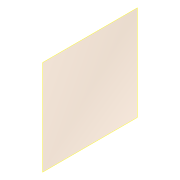
# Autodesk Inventor part: maskBodySolid
Saved by Autodesk Inventor 2018 (Build 220112000, 112)
## iProperties
Created: 2020-04-02
Part Number: maskBodySolid
Material: Generic
Document SubType Name: Modeling
Designer: Matt
Density: 1 g/cm^3
Appearance: Default
Author: Matt
Autodesk Inventor part; units mm, degrees
ref_plane "XY Plane" through (0, 0, 0) normal (0, 0, 1) x (1, 0, 0)
ref_plane "Work Plane1" through (20.32, 0, 0) normal (1, 0, 0) x (0, 1, 0)
sketch "Sketch1" plane through (20.32, 0, 0) normal (1, 0, 0) x (0, 1, 0)
  point P0 (0, 0)
sketch "Sketch2" plane through (0, 0, 0) normal (0, 0, 1) x (1, 0, 0)
  circle A0 centre (20.0816, -4.6074) radius 25.4928 projected
  point P0 (0, 0)
extrude "Extrusion1" add sketch "Sketch2" against normal blind 9.525
sketch "Sketch3" plane through (20.32, 0, 0) normal (1, 0, 0) x (0, 1, 0)
  line L0 (-30.1001, 0) -> (-30.1001, -9.525) projected
  line L1 (20.8854, 0) -> (20.8854, -9.525) projected
  line L2 (-30.1001, 0) -> (20.8854, 0) projected
  line L3 (-30.1001, 0) -> (-33.103, 5.2797) construction
  line L4 (-33.103, 5.2797) -> (-38.5488, 8.121) construction
  line L5 (-38.5488, 8.121) -> (-52.8505, 35.6829) construction
  line L6 (-52.8505, 35.6829) -> (-63.0107, 57.3273) construction
  line L7 (-63.0107, 57.3273) -> (-65.5192, 70.8376) construction
  line L8 (-65.5192, 70.8376) -> (-59.0811, 84.854) construction
  line L9 (-59.0811, 84.854) -> (-51.8304, 93.548) construction
  line L10 (-51.8304, 93.548) -> (-48.1488, 96.4774) construction
  line L11 (-48.1488, 96.4774) -> (-44.7183, 98.2529) construction
  line L12 (-44.7183, 98.2529) -> (-42.2832, 93.548) construction
  line L13 (-42.2832, 93.548) -> (-17.5193, 74.9087) construction
  line L14 (-17.5193, 74.9087) -> (7.7966, 55.4349) construction
  line L15 (7.7966, 55.4349) -> (14.1952, 48.8509) construction
  line L16 (14.1952, 48.8509) -> (14.7516, 47.2744) construction
  line L17 (14.7516, 47.2744) -> (21.4283, 26.6878) construction
  line L18 (21.4283, 26.6878) -> (28.2691, 8.9748) construction
  line L19 (28.2691, 8.9748) -> (28.2691, 1.0936) construction
  line L20 (28.2691, 1.0936) -> (28.5569, 1.0936) construction
  line L21 (28.5569, 1.0936) -> (24.3507, -0.3378) construction
  line L22 (24.3507, -0.3378) -> (20.8854, 0) construction
  spline S0 degree 4 poles (-30.1001, 0) (-33.103, 5.2797) (-38.5488, 8.121) (-52.8505, 35.6829) (-63.0107, 57.3273) (-65.5192, 70.8376) (-59.0811, 84.854) (-51.8304, 93.548) (-48.1488, 96.4774) (-44.7183, 98.2529) (-42.2832, 93.548) (-17.5193, 74.9087) (7.7966, 55.4349) (14.1952, 48.8509) (14.7516, 47.2744) (21.4283, 26.6878) (28.2691, 8.9748) (28.2691, 1.0936) (28.5569, 1.0936) (24.3507, -0.3378) (20.8854, 0) knots 1 1 1 1 1 2 3 4 5 6 7 8 9 10 11 12 13 14 15 16 17 18 18 18 18 18
  point P0 (0, 0)
  constraints: 1 perpendicular, 3 other
ref_plane "Work Plane2" through (0, 28.575, 0) normal (0, 1, 0) x (-1, 0, 0)
sketch "Sketch4" plane through (0, 28.575, 0) normal (0, 1, 0) x (-1, 0, 0)
  line L0 (-47.8363, 1.2039) -> (7.5765, 1.2039)
  point P0 (0, 0)
  constraints: 2 end point, 1 horizontal
ref_plane "Work Plane3" through (47.8363, 28.575, 1.2039) normal (0, -0.9659, -0.2588) x (-1, 0, 0)
sketch "Sketch5" plane through (47.8363, 28.575, 1.2039) normal (0, -0.9659, -0.2588) x (-1, 0, 0)
  line L0 (2.2619, -7.4253) -> (2.2619, 1.7751) projected
  line L1 (53.2475, -7.4253) -> (53.2475, 1.7751) projected
  line L2 (2.2619, -7.4253) -> (-0.1979, -10.8831) construction
  line L3 (-0.1979, -10.8831) -> (-7.0575, -19.953) construction
  line L4 (-7.0575, -19.953) -> (-10.6243, -28.0019) construction
  line L5 (-10.6243, -28.0019) -> (-13.124, -38.9334) construction
  line L6 (-13.124, -38.9334) -> (-8.1245, -54.8605) construction
  line L7 (-8.1245, -54.8605) -> (1.7075, -72.6192) construction
  line L8 (1.7075, -72.6192) -> (6.8732, -81.9495) construction
  line L9 (6.8732, -81.9495) -> (12.4542, -91.3687) construction
  line L10 (12.4542, -91.3687) -> (19.6186, -104.4781) construction
  line L11 (19.6186, -104.4781) -> (24.53, -112.0934) construction
  line L12 (24.53, -112.0934) -> (27.5166, -112.0934) construction
  ellipse E0 centre (27.7547, -7.4253) end of major axis (53.2475, -7.4253) minor radius 6.598 projected
  spline S0 degree 4 poles (2.2619, -7.4253) (-0.1979, -10.8831) (-7.0575, -19.953) (-10.6243, -28.0019) (-13.124, -38.9334) (-8.1245, -54.8605) (1.7075, -72.6192) (6.8732, -81.9495) (12.4542, -91.3687) (19.6186, -104.4781) (24.53, -112.0934) (27.5166, -112.0934) knots 1 1 1 1 1 2 3 4 5 6 7 8 9 9 9 9 9
  line L13 (27.5166, -7.5961) -> (27.5166, -11.3951)
  line L14 (52.7713, -7.4253) -> (55.2311, -10.8831) construction
  line L15 (55.2311, -10.8831) -> (62.0907, -19.953) construction
  line L16 (62.0907, -19.953) -> (65.6575, -28.0019) construction
  line L17 (65.6575, -28.0019) -> (68.1572, -38.9334) construction
  line L18 (68.1572, -38.9334) -> (63.1578, -54.8605) construction
  line L19 (63.1578, -54.8605) -> (53.3257, -72.6192) construction
  line L20 (53.3257, -72.6192) -> (48.16, -81.9495) construction
  line L21 (48.16, -81.9495) -> (42.579, -91.3687) construction
  line L22 (42.579, -91.3687) -> (35.4146, -104.4781) construction
  line L23 (35.4146, -104.4781) -> (30.5032, -112.0934) construction
  line L24 (30.5032, -112.0934) -> (27.5166, -112.0934) construction
  spline S1 degree 4 poles (52.7713, -7.4253) (55.2311, -10.8831) (62.0907, -19.953) (65.6575, -28.0019) (68.1572, -38.9334) (63.1578, -54.8605) (53.3257, -72.6192) (48.16, -81.9495) (42.579, -91.3687) (35.4146, -104.4781) (30.5032, -112.0934) (27.5166, -112.0934) knots 1 1 1 1 1 2 3 4 5 6 7 8 9 9 9 9 9
  point P0 (47.8363, -6.2329)
  constraints: 11 symmetric about line, 2 end point, 1 horizontal, 1 vertical, 7 other
body "Solid1"
